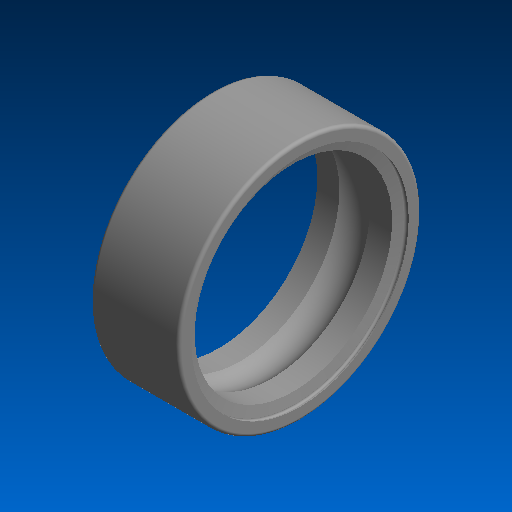
# Autodesk Inventor part: W 619/4-2Z_PART2
Saved by Autodesk Inventor 2018 (Build 220112000, 112)
## iProperties
Category: PARTsolutions
Company: SKF
Part Number: W 619/4-2Z_PART2
Material: Generic
Catalog Web Link: www.cadenas.de
Description: -Deep groove ball bearings
Vendor: SKF
Document SubType Name: Modeling
Designer: partserver
Manufacturer: SKF
Mass: 0.112633 g
Surface Area: 3.20141 cm^2
Volume: 0.112633 cm^3
Density: 1 g/cm^3
Appearance: PSOLRGB-175-175-175
PSOL_IDENT_0: {$CADENAS_DATA\23d-libs\skf\bearings_units_and_housings\ball_bearings\deep_groove_ball_bearings\bb1_
PSOL_IDENT_1: 001_101.prj},199 {VTYP=3D},{NB=W 619/4-2Z_PART2},{LINA=W 619/4-2Z_PART2},{NN=BB1_001_101_PART2},{NOP
PSOL_IDENT_2: RJ=TRUE},{DATE=06.11.2020 06:28:21},{GEOMDATE=04.11.2020 13:03:00},{VERSION=},{LINEID=15080},{WBVAR=
PSOL_IDENT_3: },{WBNUMERIC=}  {NB=W 619/4-2Z_PART2},{LINA=W 619/4-2Z_PART2},{KT=DUMMY},{DESIGNATION=W 619/4-2Z},{R
PSOL_IDENT_4: 12=0.15},{DD=4.000},{D=11.000},{B=4.000},{C=},{CX=},{CXX=},{CA=0.000},{XXVARIANT=},{XXDESIGN=Single
PSOL_IDENT_5: row stainless steel},{XXSEALING=Shield on both sides},{DESIGN=dgbbw2z},{VARIANT=},{DD1=6.15},{DD2=5.
PSOL_IDENT_6: 6},{DD2X=},{DD2A=5.60},{D1=8.95},{D1X=MIN},{D2=9.85},{D2A=9.85},{D3=},{D3X=},{D3A=0.000},{D4=},{HH=M
PSOL_IDENT_7: IN},{BB=},{BBX=},{BBA=0.000},{FF=},{R0MAX=MIN},{R0=MIN},{PITCH=7.51},{DW=2.000},{DDAMIN=5.200},{DDAM
PSOL_IDENT_8: AX=5.500},{DDBMIN=MIN},{DDBMAX=MIN},{DBMIN=MIN},{DAMAX=10.000},{BBAMIN=MIN},{CAMAX=MIN},{RAMAX=0.150
PSOL_IDENT_9: },{LOAD1=0.540},{LOAD2=0.176},{LOAD3=0.008},{SPEED1=130000},{SPEED2=63000},{KR=0.025},{F0=6.400},{Z=
PSOL_IDENT_10: 7},{II=1},{MASS=0.002},{BEARING=W 619/4-2Z},{RING=},{HELP=1.025},{HELP2=0.575},{DD1ALG=3.075},{YALG=
PSOL_IDENT_11: 3.075},{PITCH1=7.510},{DW1=2.000},{YALG1=4.475},{HALG1=1.025},{SH=2.800},{CU=0.400},{HALG=1.075},{B1=
PSOL_IDENT_12: 0},{SHIELDHELP=2},{D4A=0.000},{FFA=0.000},{RS1=}
NB: W 619/4-2Z_PART2
NT: Deep groove ball bearings
NBSYN: $DESIGNATION._PART2
LINA: W 619/4-2Z_PART2
CATALOG: SKF
SUPPLIER: SKF
ARTICLENO: W 619/4-2Z_PART2
BOMINFO: W 619/4-2Z_PART2
CREATOR: CADENAS GmbH
Title: W 619/4-2Z_PART2
Author: Cadenas PARTsolutions
Comments: Deep groove ball bearings
Autodesk Inventor part; units mm, degrees
ref_plane "YZ Plane" through (0, 0, 0) normal (1, 0, 0) x (0, 1, 0)
ref_plane "XZ Plane" through (0, 0, 0) normal (0, 1, 0) x (-1, 0, 0)
ref_plane "XY Plane" through (0, 0, 0) normal (0, 0, 1) x (1, 0, 0)
sketch "Sketch_17" plane through (0, 0, 0) normal (0, 0, 1) x (1, 0, 0)
  line L0 (50, 0) -> (-50, 0)
  line L1 (0, 5.35) -> (0, 4.925)
  line L2 (0, 4.925) -> (0.045, 4.925)
  arc A0 (0.225, 4.925) -> (0.045, 4.925) centre (0.135, 4.925) ccw
  line L3 (0.225, 4.925) -> (0.3043, 4.475)
  line L4 (0.3043, 4.475) -> (1.306, 4.475)
  arc A1 (2.694, 4.475) -> (1.306, 4.475) centre (2, 3.755) ccw
  line L5 (2.694, 4.475) -> (3.6957, 4.475)
  line L6 (3.6957, 4.475) -> (3.775, 4.925)
  arc A2 (3.955, 4.925) -> (3.775, 4.925) centre (3.865, 4.925) ccw
  line L7 (3.955, 4.925) -> (4, 4.925)
  line L8 (4, 4.925) -> (4, 5.35)
  arc A3 (4, 5.35) -> (3.85, 5.5) centre (3.85, 5.35) ccw
  line L9 (3.85, 5.5) -> (0.15, 5.5)
  arc A4 (0.15, 5.5) -> (0, 5.35) centre (0.15, 5.35) ccw
  constraints: 20 end point, 10 point on circle, 5 centre point
revolve "Revolution1" add sketch "Sketch_17" angle 360 about axis through (50, 0, 0) along (1, 0, 0)
body "Solid1"
